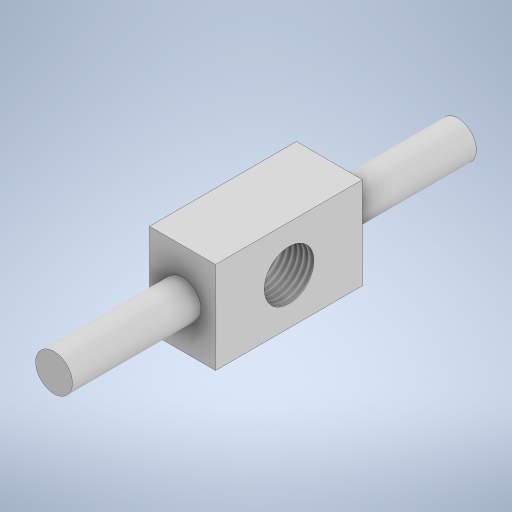
# Autodesk Inventor part: sworzeń z nakrętką
Saved by Autodesk Inventor 2024 (Build 280153000, 153)
## iProperties
Created: 2024-09-19
Part Number: sworzeń z nakrętką
Material: Ogólny
Document SubType Name: Modeling
Designer: JEDEN
Density: 1 g/cm^3
Appearance: Domyślna
Author: JEDEN
Autodesk Inventor part; units mm, degrees
ref_plane "YZ Plane" through (0, 0, 0) normal (1, 0, 0) x (0, 1, 0)
ref_plane "XZ Plane" through (0, 0, 0) normal (0, 1, 0) x (-1, 0, 0)
ref_plane "XY Plane" through (0, 0, 0) normal (0, 0, 1) x (1, 0, 0)
sketch "Szkic1" plane through (0, 0, 0) normal (0, 0, 1) x (1, 0, 0)
  line L0 (-18.8999, 4.9578) -> (17.1001, 4.9578)
  line L1 (17.1001, 4.9578) -> (17.1001, -45.0422)
  line L2 (17.1001, -45.0422) -> (-18.8999, -45.0422)
  line L3 (-18.8999, -45.0422) -> (-18.8999, 4.9578)
  point P0 (0, 0)
  dimension "d0" = 36
  dimension "d1" = 50
  constraints: 8 end point, 2 parallel, 1 horizontal, 1 perpendicular
  measures "d0" distance of L1.end L2.end
  measures "d1" distance of L0.end L1.end
extrude "Wyciągnięcie proste1" add sketch "Szkic1" along normal blind 40
sketch "Szkic2" plane through (0, 0, 40) normal (0, 0, 1) x (1, 0, 0)
  line L0 (-18.8999, 4.9578) -> (-18.8999, -45.0422) projected
  line L1 (-18.8999, -45.0422) -> (17.1001, -45.0422) projected
  line L2 (-18.8999, 4.9578) -> (17.1001, -45.0422)
  line L3 (17.1001, -45.0422) -> (17.1001, 4.9578) projected
  line L4 (17.1001, 4.9578) -> (-18.8999, -45.0422)
  circle A0 centre (-0.8999, -20.0422) radius 10
  point P0 (0, 0)
  dimension "d4" = 20
  constraints: 4 end point, 1 centre point, 1 midpoint
  measures "d4" diameter of A0
extrude "Wyciągnięcie proste2" add sketch "Szkic2" along normal blind 70 contours A0 L4 L2 | L2 L4 A0 | L4 L2 A0 | L4 A0 L2
mirror "Odbij1" about plane through (-0.8999, -20.0422, 0) normal (0, 0, -1)
sketch "Szkic3" plane through (17.1001, -45.0422, 40) normal (1, 0, 0) x (0, 0, -1)
  line L0 (0, 0) -> (0, 50) projected
  line L1 (80, 0) -> (0, 0) projected
  line L2 (0, 50) -> (80, 0)
  line L3 (80, 0) -> (80, 50) projected
  line L4 (80, 50) -> (0, 0)
  point P0 (40, 45.0422)
  point P1 (40, 25)
  constraints: 4 end point, 1 midpoint
hole "Otwór1" at (17.1001, -20.0422, 0) direction (-1, 0, 0) diameter 27 end through all thread size "TR30x3" class "7H" standard "ISO Metric Trapezoidal Threads"
